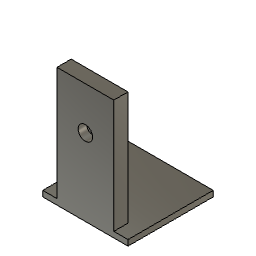
Detector_Holder (Autodesk Fusion 360 design; units mm, degrees)
Autodesk Fusion 360 part; units mm, degrees
sketch "Sketch1" plane through (0, 0, 0) normal (0, 0, 1) x (1, 0, 0)
  line L0 (15, -15) -> (-15, -15)
  line L1 (-15, -15) -> (-15, 15)
  line L2 (-15, 15) -> (15, 15)
  line L3 (15, 15) -> (15, -15)
  line L4 (15, -15) -> (-15, 15) construction
  line L5 (-15, -15) -> (15, 15) construction
  dimension "d1" = 30
  dimension "d2" = 30
  constraint horizontal L0
  constraint perpendicular L0 L1
  constraint parallel L0 L2
  constraint parallel L1 L3
  constraint coincident L4 origin
  constraint coincident L5 origin
  measures "d1" distance of L1.end L2.end
  measures "d2" distance of L0.end L1.end
extrude "Extrude1" add sketch "Sketch1" along normal blind 2 makes body 1
sketch "Sketch2" plane through (0, 0, 2) normal (0, 0, 1) x (-1, 0, 0)
  line L0 (-15, -15) -> (15, -15)
  line L1 (15, -15) -> (15, 15)
  line L2 (15, 15) -> (-15, 15)
  line L3 (-15, 15) -> (-15, -15)
  line L4 (15, 15) -> (10, 15) construction
  line L5 (10, 15) -> (10, 10) construction
  line L6 (10, 10) -> (15, 10) construction
  line L7 (15, 10) -> (15, 15) construction
  line L8 (-15, 15) -> (-10, 15) construction
  line L9 (-10, 15) -> (-10, 10) construction
  line L10 (-10, 10) -> (-15, 10) construction
  line L11 (-15, 10) -> (-15, 15) construction
  line L12 (10, 15) -> (-10, 15)
  line L13 (-10, 15) -> (-10, 10)
  line L14 (-10, 10) -> (10, 10)
  line L15 (10, 10) -> (10, 15)
  dimension "d5" = 5
  dimension "d6" = 5
  dimension "d7" = 5
  dimension "d8" = 5
  constraint horizontal L4
  constraint vertical L5
  constraint horizontal L6
  constraint vertical L7
  constraint coincident L1.end L2.start
  constraint horizontal L8
  constraint vertical L9
  constraint horizontal L10
  constraint vertical L11
  constraint coincident L2.end L3.start
  constraint horizontal L12
  constraint vertical L13
  constraint horizontal L14
  constraint vertical L15
  measures "d5" distance of L1.end L4.end
  measures "d6" distance of L1.end L6.end
  measures "d7" distance of L2.end L8.end
  measures "d8" distance of L2.end L10.end
extrude "Extrude2" add sketch "Sketch2" along normal blind 40 contours L2 L12 L13 L14 L15 bodies 1
sketch "Sketch3" plane through (0, -15, 0) normal (0, -1, 0) x (1, 0, 0)
  line L0 (-15, 0) -> (15, 0)
  line L1 (15, 0) -> (15, 2)
  line L2 (15, 2) -> (10, 2)
  line L3 (10, 2) -> (10, 42)
  line L4 (10, 42) -> (-10, 42)
  line L5 (-10, 42) -> (-10, 2)
  line L6 (-10, 2) -> (-15, 2)
  line L7 (-15, 2) -> (-15, 0)
  line L8 (10, 2) -> (0, 2) construction
  line L9 (0, 2) -> (0, 27) construction
  line L10 (0, 27) -> (10, 27) construction
  line L11 (10, 27) -> (10, 2) construction
  circle A0 centre (0, 27) radius 2.55
  dimension "d11" = 10
  dimension "d12" = 25
  dimension "d13" = 5.1
  constraint horizontal L8
  constraint vertical L9
  constraint horizontal L10
  constraint vertical L11
  constraint coincident L2.end L3.start
  constraint coincident L9.end L10.start
  measures "d11" distance of L2.end L8.end
  measures "d12" distance of L2.end L10.end
  measures "d13" diameter of A0
sketch "Sketch4" plane through (0, -15, 0) normal (0, -1, 0) x (1, 0, 0)
  line L0 (-15, 0) -> (15, 0)
  line L1 (15, 0) -> (15, 2)
  line L2 (15, 2) -> (10, 2)
  line L3 (10, 2) -> (10, 42)
  line L4 (10, 42) -> (-10, 42)
  line L5 (-10, 42) -> (-10, 2)
  line L6 (-10, 2) -> (-15, 2)
  line L7 (-15, 2) -> (-15, 0)
  line L8 (0, 27) -> (1.75, 27) construction
  line L9 (0, 27) -> (-1.75, 27) construction
  circle A0 centre (1.75, 27) radius 0.5
  circle A1 centre (-1.75, 27) radius 0.5
  point P0 (0, 27)
  dimension "d14" = 1.75
  dimension "d15" = 1.75
  dimension "d16" = 1
  dimension "d17" = 1
  constraint horizontal L8
  constraint coincident P0 L8.start
  constraint coincident L8.end A0.centre
  constraint coincident L9.end A1.centre
  measures "d14" distance of P0 L8.end
  measures "d15" distance of P0 L9.end
  measures "d16" diameter of A0
  measures "d17" diameter of A1
extrude "Extrude3" cut sketch "Sketch4" against normal up to surface (5 mm away) contours A0 | A1 bodies 1
extrude "Extrude4" cut sketch "Sketch3" against normal blind 3 contours A0 bodies 1
copy_body "Body->Comp1" bodies 1 removing the originals makes body 2 in component "Detector_Holder"
component "Detector_Holder" placed x (1, 0, 0) y (0, 1, 0) z (0, 0, 1) at (0, 0, 0)
